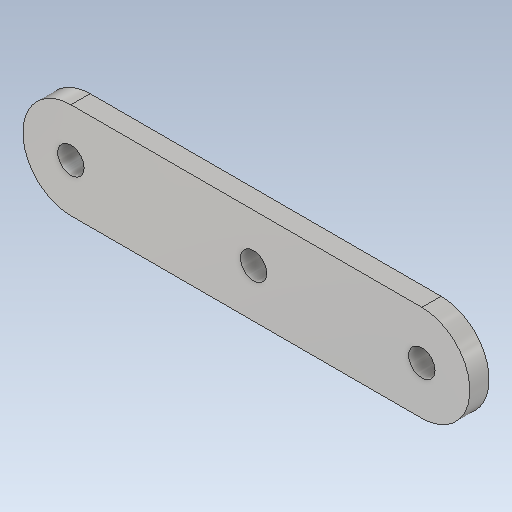
# Autodesk Inventor part: encoder_link
Saved by Autodesk Inventor 2020 (Build 240168000, 168)
## iProperties
Created: 2017-11-27
Part Number: encoder_link
Material: Generic
Document SubType Name: Modeling
Designer: stedrock
Density: 1 g/cm^3
Appearance: Default
Mass: 6.81154 g
Surface Area: 44.4844 cm^2
Volume: 6.81154 cm^3
Author: stedrock
Autodesk Inventor part; units mm, degrees
ref_plane "YZ Plane" through (0, 0, 0) normal (1, 0, 0) x (0, 1, 0)
ref_plane "XZ Plane" through (0, 0, 0) normal (0, 1, 0) x (-1, 0, 0)
ref_plane "XY Plane" through (0, 0, 0) normal (0, 0, 1) x (1, 0, 0)
sketch "Sketch1" plane through (0, 0, 0) normal (0, 0, 1) x (1, 0, 0)
  line L0 (-46.5, -10) -> (46.5, -10)
  line L1 (46.5, -10) -> (46.5, 10)
  line L2 (46.5, 10) -> (-46.5, 10)
  line L3 (-46.5, 10) -> (-46.5, -10)
  line L4 (-46.5, -10) -> (46.5, 10) construction
  line L5 (46.5, -10) -> (-46.5, 10) construction
  line L6 (0, 0) -> (-57.93, 0) construction
  circle A0 centre (-36.5, 0) radius 2.75
  line L7 (0, 0) -> (0, 23.3519) construction
  circle A1 centre (36.5, 0) radius 2.75
  circle A2 centre (1.5, 0) radius 2.75
  dimension "d0" = 93
  dimension "d1" = 20
  dimension "d5" = 5.5
  dimension "d6" = 10
  dimension "d9" = 5.5
  dimension "d11" = 35
  constraints: 16 end point, 3 centre point, 2 equal length, 2 midpoint, 2 point on line, 2 vertical, 1 horizontal, 1 parallel, 1 symmetric about line, 1 other
  measures "d0" distance of L2.end L1.end
  measures "d1" distance of L1.end L0.end
  measures "d5" diameter of A0
  measures "d6" distance from line of L3 A0.centre
  measures "d9" diameter of A2
  measures "d11" distance of A1.centre A2.centre
extrude "Extrusion1" add sketch "Sketch1" along normal blind 4 contours L3 L2 L1 L0 | A0 | A1 | A2
fillet "Fillet1" radius 10 4 edges at (-46.5, 10, 2) (-46.5, -10, 2) (46.5, 10, 2) (46.5, -10, 2)
extrude "Extrusion2" cut sketch "Sketch1" along normal through all contours A0 | A1 | A2
equation "\"d9\" = d5"
body "Solid1"
